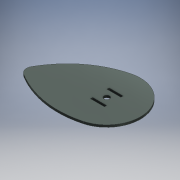
# Autodesk Inventor part: leva00
Saved by Autodesk Inventor 2016 (Build 200138000, 138)
## iProperties
Created: 2016-09-20
Part Number: leva00
Material: Madera (abedul)
Document SubType Name: Modeling
Designer: i95sa
Density: 0.55 g/cm^3
Appearance: Gris plomo - Pulido
Author: i95sa
Autodesk Inventor part; units mm, degrees
ref_plane "YZ Plane" through (0, 0, 0) normal (1, 0, 0) x (0, 1, 0)
ref_plane "XZ Plane" through (0, 0, 0) normal (0, 1, 0) x (-1, 0, 0)
ref_plane "XY Plane" through (0, 0, 0) normal (0, 0, 1) x (1, 0, 0)
sketch "Boceto1" plane through (0, 0, 0) normal (0, 0, 1) x (1, 0, 0)
  arc A0 (57.6694, 14.807) -> (-57.6694, -14.807) centre (0, 0) ccw
  arc A1 (-88.7487, -22.7868) -> (-115.3654, -29.6208) centre (-102.0571, -26.2038) ccw
  line L0 (-119.2185, -30.6101) -> (-122.6355, -17.3018)
  line L1 (-14.1228, 57.8408) -> (-19.8178, 80.0214)
  line L2 (-19.8178, 80.0214) -> (-122.6355, -17.3018)
  line L3 (-122.6355, -17.3018) -> (-82.721, 20.4797)
  arc A2 (-14.1228, 57.8408) -> (-82.721, 20.4797) centre (22.0169, -90.1714) ccw
  arc A3 (-82.721, 20.4797) -> (-114.0004, -19.4109) centre (35.5518, -104.4705) ccw
  line L4 (4.4361, 1.139) -> (57.6694, 14.807)
  line L5 (-4.4361, -1.139) -> (-119.2185, -30.6101)
  arc A4 (-57.6694, -14.807) -> (57.6694, 14.807) centre (0, 0) ccw
  arc A5 (-115.3654, -29.6208) -> (-88.7487, -22.7868) centre (-102.0571, -26.2038) ccw
  line L6 (-119.2185, -30.6101) -> (-115.8015, -43.9184)
  line L7 (15.4891, -57.49) -> (21.1841, -79.6705)
  line L8 (21.1841, -79.6705) -> (-115.8015, -43.9184)
  line L9 (-115.8015, -43.9184) -> (-62.6228, -57.7976)
  arc A6 (-62.6228, -57.7976) -> (15.4891, -57.49) centre (-24.1469, 89.6246) ccw
  arc A7 (-109.2506, -37.9102) -> (-62.6228, -57.7976) centre (-19.1748, 108.6754) ccw
  dimension "d0" = 119.08
  dimension "d6" = 27.48
  dimension "d7" = 13.74
  dimension "d8" = 22.9
  dimension "d9" = 54.96
  constraints: 20 end point, 20 point on circle, 8 centre point, 6 symmetric about line, 5 point on line, 4 tangent, 1 collinear, 4 other
  measures "d0" diameter of A0
  measures "d6" diameter of A1
  measures "d7" distance of L0.start L0.end
  measures "d8" distance of L1.start L1.end
  measures "d9" distance of L0.end L3.end
extrude "Extrusión2" add sketch "Boceto1" along normal blind 4 contours A4 A0 | A0 L5 A1 A3 A2 | A6 A7 A5 L5 A4 | L5 A1 | A5 L5
sketch "Boceto2" plane through (0, 0, 4) normal (0, 0, 1) x (1, 0, 0)
  line L0 (0, 0) -> (0, 12.5)
  line L1 (0, 12.5) -> (-12.5, 12.5)
  line L2 (-12.5, 12.5) -> (-12.5, 16.7)
  line L3 (-12.5, 16.7) -> (12.5, 16.7)
  line L4 (12.5, 16.7) -> (12.5, 12.5)
  line L5 (12.5, 12.5) -> (0, 12.5)
  line L6 (0, 0) -> (12.5, 0)
  line L7 (0, 0) -> (0, -12.5)
  line L8 (0, -12.5) -> (-12.5, -12.5)
  line L9 (-12.5, -12.5) -> (-12.5, -16.7)
  line L10 (-12.5, -16.7) -> (12.5, -16.7)
  line L11 (12.5, -16.7) -> (12.5, -12.5)
  line L12 (12.5, -12.5) -> (0, -12.5)
  circle A0 centre (0, 0) radius 5
  dimension "d24" = 12.5
  dimension "d25" = 12.5
  dimension "d26" = 4.2
  dimension "d27" = 25
  dimension "d28" = 10
  constraints: 26 end point, 5 perpendicular, 5 symmetric about line, 3 point on line, 1 centre point, 1 coincident, 1 parallel, 1 vertical
  measures "d24" distance of L0.start L0.end
  measures "d25" distance of L0.end L1.end
  measures "d26" distance of L1.end L2.end
  measures "d27" distance of L2.end L3.end
  measures "d28" diameter of A0
extrude "Extrusión3" cut sketch "Boceto2" against normal blind 4
